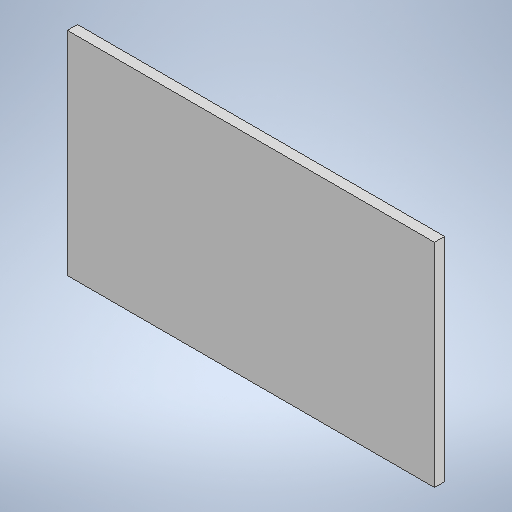
# Autodesk Inventor part: Part2
Saved by Autodesk Inventor 2025.1 (Build 291241000, 241)
## iProperties
Created: 2024-12-01
Part Number: Part2
Material: Generic
Document SubType Name: Modeling
Designer: Cristhian Vigo
Density: 1 g/cm^3
Appearance: Default
Author: Cristhian Vigo
Autodesk Inventor part; units mm, degrees
ref_plane "YZ Plane" through (0, 0, 0) normal (1, 0, 0) x (0, 1, 0)
ref_plane "XZ Plane" through (0, 0, 0) normal (0, 1, 0) x (-1, 0, 0)
ref_plane "XY Plane" through (0, 0, 0) normal (0, 0, 1) x (1, 0, 0)
sketch "Sketch1" plane through (0, 0, 0) normal (0, 0, 1) x (1, 0, 0)
  line L0 (-22.987, 13.2969) -> (22.987, 13.2969)
  line L1 (22.987, 13.2969) -> (22.987, -13.2969)
  line L2 (22.987, -13.2969) -> (-22.987, -13.2969)
  line L3 (-22.987, -13.2969) -> (-22.987, 13.2969)
  point P0 (0, 0)
  point P1 (0, -13.2969)
  point P2 (22.987, 0)
  dimension "d0" = 45.974
  dimension "d1" = 26.5938
  constraints: 8 end point, 2 midpoint, 2 parallel, 1 horizontal, 1 horizontal alignment, 1 perpendicular, 1 vertical alignment
  measures "d0" distance of L1.end L2.end
  measures "d1" distance of L0.end L1.end
extrude "Extrusion1" add sketch "Sketch1" along normal blind 1.27
body "Solid1"
